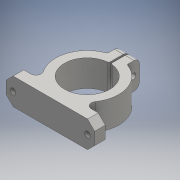
# Autodesk Inventor part: atomizer_holder
Saved by Autodesk Inventor 2016 (Build 200138000, 138)
## iProperties
Created: 2016-10-21
Part Number: atomizer_holder
Material: Generic
Document SubType Name: Modeling
Designer: rawrdong
Density: 1 g/cm^3
Appearance: Default
Author: rawrdong
Autodesk Inventor part; units mm, degrees
ref_plane "YZ Plane" through (0, 0, 0) normal (1, 0, 0) x (0, 1, 0)
ref_plane "XZ Plane" through (0, 0, 0) normal (0, 1, 0) x (-1, 0, 0)
ref_plane "XY Plane" through (0, 0, 0) normal (0, 0, 1) x (1, 0, 0)
sketch "Sketch1" plane through (0, 0, 0) normal (0, 0, 1) x (1, 0, 0)
  line L0 (0, 0) -> (25, 0)
  line L1 (25, 0) -> (25, 6)
  line L2 (25, 6) -> (17.1289, 6)
  arc A0 (14.6584, 10.7019) -> (5.5, 37.729) centre (0, 20.8) ccw
  line L3 (0, 0) -> (0, 8)
  arc A1 (0, 8) -> (0.5, 33.5902) centre (0, 20.8) ccw
  arc A2 (14.6584, 10.7019) -> (17.1289, 6) centre (17.1289, 9) ccw
  line L4 (5.5, 37.729) -> (5.5, 44.729)
  line L5 (5.5, 44.729) -> (0.5, 44.729)
  line L6 (0.5, 44.729) -> (0.5, 33.5902)
  point P0 (9.8894, 6)
  dimension "d0" = 12.8
  dimension "d2" = 5
  dimension "d3" = 25
  dimension "d4" = 6
  dimension "d5" = 8
  dimension "d6" = 3
  dimension "d7" = 1
  dimension "d8" = 5
  dimension "d9" = 7
  constraints: 14 end point, 7 point on circle, 4 perpendicular, 3 centre point, 2 tangent, 2 vertical, 1 coincident, 1 horizontal, 1 point on line, 1 vertical alignment
  measures "d0" radius of A1
  measures "d2" radial gap between concentric circles of A0 A1
  measures "d3" distance of L0.start L0.end
  measures "d4" distance between parallel lines of L0 L2
  measures "d5" distance of L0.start L3.end
  measures "d6" radius of A2
  measures "d7" diameter of L6 L3
  measures "d8" distance between parallel lines of L4 L6
  measures "d9" distance of L4.start L4.end
extrude "Extrusion1" add sketch "Sketch1" along normal blind 15
sketch "Sketch2" plane through (17.1289, 6, 0) normal (0, 1, 0) x (1, 0, 0)
  line L0 (7.8711, 0) -> (7.8711, -15) projected
  line L1 (7.8711, -15) -> (0, 0) construction
  line L2 (7.8711, 0) -> (0, 0) projected
  circle A0 centre (3.9355, -7.5) radius 1.6
  point P0 (-17.1289, 0)
  dimension "d15" = 3.2
  constraints: 2 end point, 1 centre point, 1 midpoint
  measures "d15" diameter of A0
extrude "Extrusion2" cut sketch "Sketch2" against normal through all
chamfer "Chamfer1" distance 4 angle 45 2 edges at (25, 3, 15) (25, 3, 0)
sketch "Sketch3" plane through (5.5, 37.729, 0) normal (1, 0, 0) x (0, 0, -1)
  line L0 (-15, 0) -> (0, 7) construction
  point P0 (0, -37.729)
  point P1 (-7.5, 3.5)
  constraints: 2 end point, 1 midpoint
hole "Hole1" at (5.5, 41.229, 7.5) direction (-1, 0, 0) diameter 3.2 end through all
fillet "Fillet1" radius 3 2 edges at (3, 44.729, 0) (3, 44.729, 15)
fillet "Fillet1" radius 1 2 edges at (5.5, 37.729, 7.5) (0.5, 33.5902, 7.5)
mirror "Mirror1" about plane through (0, 8, 0) normal (-1, 0, 0)
body "Solid1"
